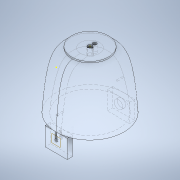
# Autodesk Inventor part: EnclosingRevolver
Saved by Autodesk Inventor 2021.1 (Build 251245010, 245A)
## iProperties
Created: 2023-07-02
Part Number: EnclosingRevolver
Material: ABS Plastic
Document SubType Name: Modeling
Designer: Drake
Density: 1.06 g/cm^3
Appearance: Smooth - White
Author: Drake
Autodesk Inventor part; units mm, degrees
ref_plane "XZ Plane" through (0, 0, 0) normal (0, 1, 0) x (-1, 0, 0)
sketch "Sketch1" plane through (0, 0, 0) normal (0, 1, 0) x (-1, 0, 0)
  arc A0 (-5.4792, -2.4451) -> (-5.4792, 2.4451) centre (0, 0) ccw
  circle A1 centre (0, 0) radius 50
  line L0 (0, 0) -> (0, 6.8)
  circle A2 centre (0, 6.8) radius 0.75
  arc A3 (-5.4792, 2.4451) -> (-5.4792, -2.4451) centre (-6, 0) ccw
  dimension "crescenttop" = 12
  dimension "pantiltmotorholderdiam" = 100
  dimension "screwhole" = 6.8
  dimension "screwhole2" = 1.5
  dimension "CorrectedCrescent" = 5
  constraints: 5 point on circle, 4 centre point, 3 coincident, 2 end point, 1 vertical
  measures "crescenttop" diameter of A0
  measures "pantiltmotorholderdiam" diameter of A1
  measures "screwhole" distance of L0.start L0.end
  measures "screwhole2" diameter of A2
  measures "CorrectedCrescent" diameter of A3
extrude "Extrusion1" add sketch "Sketch1" along normal blind 3.7
ref_plane "Work Plane2" through (-25, 0, 0) normal (1, 0, 0) x (0, 1, 0)
ref_plane "Work Plane1" through (25, 0, 0) normal (1, 0, 0) x (0, 1, 0)
sketch "Sketch3" plane through (0, 0, 0) normal (1, 0, 0) x (0, 1, 0)
  line L0 (0, 25.8902) -> (0, 82.1004) construction
  line L1 (0, 82.1004) -> (-19.2329, 82.1004) construction
  line L2 (-19.2329, 82.1004) -> (-150.2459, 92.0453) construction
  line L3 (-150.2459, 92.0453) -> (-151.1107, 92.0453) construction
  spline S0 degree 4 poles (0, 25.8902) (0, 82.1004) (-19.2329, 82.1004) (-150.2459, 92.0453) (-151.1107, 92.0453) knots 1 1 1 1 1 2 2 2 2 2
  line L4 (0, -50) -> (0, 50) projected
  line L5 (-151.1107, 92.0453) -> (-151.1107, 77.0453)
  line L6 (-151.1107, 77.0453) -> (-80.8125, 71.4468) construction
  line L7 (-80.8125, 71.4468) -> (-20.5383, 53.8321) construction
  line L8 (-20.5383, 53.8321) -> (-22.6717, 53.8321) construction
  line L9 (-22.6717, 53.8321) -> (-15, 0) construction
  spline S1 degree 4 poles (-151.1107, 77.0453) (-80.8125, 71.4468) (-20.5383, 53.8321) (-22.6717, 53.8321) (-15, 0) knots 1 1 1 1 1 2 2 2 2 2
  line L10 (0, 50) -> (0, 0)
  line L11 (0, 50) -> (0, 0)
  line L12 (-15, -28.9058) -> (-15, -27.5917)
  line L13 (0, 25.8902) -> (0, -27.5917)
  line L14 (-15, 0) -> (0, 0)
  dimension "d9" = 15
  dimension "d10" = 15
  constraints: 12 end point, 3 horizontal, 2 point on line, 2 vertical, 1 collinear, 1 parallel, 6 other
  measures "d9" distance of L10.end L9.end
  measures "d10" distance of L3.end L5.end
revolve "Revolution1" add sketch "Sketch3" angle 360 about axis through (0, -15, 0) along (0, -1, 0)
mirror "Mirror1" about plane through (0, 0, 0) normal (0, 0, 1) of "Revolution1"
ref_plane "Work Plane3" through (0, 0, 92.0455) normal (0, 0, 1) x (1, 0, 0)
sketch "Sketch4" plane through (0, 0, 92.0455) normal (0, 0, 1) x (1, 0, 0)
  line L0 (-92.0453, -151.1107) -> (92.0453, -151.1107) projected
  line L1 (-92.0453, -151.1107) -> (-92.0453, -139.1107)
  line L2 (-92.0453, -151.1107) -> (-92.0453, -118.1107)
  line L3 (-92.0453, -118.1107) -> (-92.0453, -113.1107)
  line L4 (-92.0453, -113.1107) -> (0, -113.1107)
  point P0 (0, 0)
  point P1 (0, -151.1107)
  dimension "motorwidth" = 12
  dimension "motorlength" = 33
  dimension "allowance" = 5
  constraints: 8 end point, 3 vertical, 1 coincident, 1 perpendicular
  measures "motorwidth" distance of L0.start L1.end
  measures "motorlength" distance of L0.start L2.end
  measures "allowance" distance of L2.end L3.end
hole "Hole1" at (0, -113.1107, 92.0455) direction (0, 0, -1) diameter 3 end through all
thread "Thread1" size "M3x0.5" class "6H" standard "ANSI Metric M Profile" full length
sketch "Sketch6" plane through (0, -151.1107, 0) normal (0, -1, 0) x (1, 0, 0)
  circle A0 centre (0, 0) radius 92.0453 projected
  circle A1 centre (0, 0) radius 77.0453
  circle A2 centre (0, 0) radius 77.0453 projected
  line L0 (0, -77.0453) -> (25, -77.0453)
  line L1 (25, -77.0453) -> (30, -77.0453)
  line L2 (30, -77.0453) -> (-25, -77.0453)
  line L3 (-25, -77.0453) -> (-30, -77.0453)
  line L4 (-30, -77.0453) -> (-30, -79.5453)
  line L5 (-30, -79.5453) -> (-30, -91.5453)
  line L6 (-30, -91.5453) -> (30, -91.5453)
  line L7 (30, -91.5453) -> (30, -77.0453)
  line L8 (-30, -77.0453) -> (-30, -81.0453)
  point P0 (0, 77.0453)
  point P1 (-4.9974, -76.883)
  point P2 (-4.9974, -91.9095)
  point P3 (0, 92.0453)
  point P4 (4.9974, -91.9095)
  point P5 (-30, -87.0191)
  point P6 (-9.581, -91.5453)
  point P7 (9.581, -91.5453)
  point P8 (30, -87.0191)
  dimension "d43" = 25
  dimension "d44" = 5
  dimension "d45" = 55
  dimension "d46" = 5
  dimension "supportwidth" = 60
  dimension "bushingpenetration" = 2.5
  dimension "d49" = 12
  dimension "d50" = 0
  dimension "d51" = 14.5
  dimension "bushinglength" = 4
  dimension "d60" = 14.5
  constraints: 18 end point, 4 point on line, 3 point on circle, 1 coincident, 1 horizontal, 1 perpendicular, 1 tangent, 1 vertical, 3 other
  measures "d43" distance of L0.start L0.end
  measures "d44" distance of L0.end L1.end
  measures "d45" distance of L1.end L2.end
  measures "d46" distance of L2.end L3.end
  measures "supportwidth" distance of L1.end L3.end
  measures "bushingpenetration" distance of L3.end L4.end
  measures "d49" distance of L4.end L5.end
  measures "d50" angle of L6 L3
  measures "d51" distance from line of L5.end L3
  measures "bushinglength" distance of L3.end L8.end
  measures "d60" distance of L6.end L1.end
extrude "Extrusion2" add sketch "Sketch6" along normal blind 50 contours L5 L4 L3 L2 L0 L1 L7 A0 L6 | A0 L6 L5 | L7 L6 A0
mirror "Mirror2" about plane through (0, 0, 0) normal (0, 0, 1) of "Extrusion2"
sketch "Sketch8" plane through (0, 3.7, 0) normal (0, 1, 0) x (1, 0, 0)
  arc A0 (5.4792, 2.4451) -> (5.4792, -2.4451) centre (0, 0) ccw construction
  line L0 (0, 0) -> (0, 25) construction
  circle A1 centre (0, 0) radius 25 construction
  circle A2 centre (0, 12.5) radius 5
  line L1 (0, 0) -> (0, -6.8)
  circle A3 centre (0, -6.8) radius 0.75
  point P0 (-6, 0)
  point P1 (-6, 0)
  point P2 (-1.4882, 5.8125)
  point P3 (1.4882, 5.8125)
  dimension "d40" = 10
  dimension "d56" = 6.8
  dimension "d57" = 1.5
  constraints: 4 end point, 2 centre point, 2 vertical, 1 coincident, 1 midpoint, 1 vertical alignment, 1 other
  measures "d40" diameter of A2
  measures "d56" distance of L1.start L1.end
  measures "d57" diameter of A3
extrude "Extrusion4" cut sketch "Sketch8" against normal through all
sketch "Sketch9" plane through (0, 3.7, 0) normal (0, 1, 0) x (1, 0, 0)
  point P0 (0, 0)
ref_plane "Work Plane4" through (0, -171.1107, 92.0455) normal (0, 0, 1) x (1, 0, 0)
sketch "Sketch10" plane through (0, -171.1107, 92.0455) normal (0, 0, 1) x (1, 0, 0)
  line L0 (-1.9, 16.6) -> (-2.75, 2.1651)
  line L1 (2.75, 2.1651) -> (1.9, 16.6)
  arc A0 (1.9, 16.6) -> (-1.9, 16.6) centre (0, 16.6) ccw
  circle A1 centre (0, 0) radius 3.5
  circle A2 centre (0, 0) radius 1.25
  line L2 (0.6339, 2.1589) -> (0.3485, 2.4241)
  line L3 (0.3485, 2.4241) -> (0, 2.25)
  line L4 (0, 2.25) -> (-0.3485, 2.4241)
  line L5 (-0.3485, 2.4241) -> (-0.6339, 2.1589)
  line L6 (-0.6339, 2.1589) -> (-1.0174, 2.2278)
  line L7 (-1.0174, 2.2278) -> (-1.2164, 1.8928)
  line L8 (-1.2164, 1.8928) -> (-1.6038, 1.8509)
  line L9 (-1.6038, 1.8509) -> (-1.7004, 1.4734)
  line L10 (-1.7004, 1.4734) -> (-2.0603, 1.3241)
  line L11 (-2.0603, 1.3241) -> (-2.0467, 0.9347)
  line L12 (-2.0467, 0.9347) -> (-2.3499, 0.69)
  line L13 (-2.3499, 0.69) -> (-2.2271, 0.3202)
  line L14 (-2.2271, 0.3202) -> (-2.4491, 0)
  line L15 (-2.4491, 0) -> (-2.2271, -0.3202)
  line L16 (-2.2271, -0.3202) -> (-2.3499, -0.69)
  line L17 (-2.3499, -0.69) -> (-2.0467, -0.9347)
  line L18 (-2.0467, -0.9347) -> (-2.0603, -1.3241)
  line L19 (-2.0603, -1.3241) -> (-1.7004, -1.4734)
  line L20 (-1.7004, -1.4734) -> (-1.6038, -1.8509)
  line L21 (-1.6038, -1.8509) -> (-1.2164, -1.8928)
  line L22 (-1.2164, -1.8928) -> (-1.0174, -2.2278)
  line L23 (-1.0174, -2.2278) -> (-0.6339, -2.1589)
  line L24 (-0.6339, -2.1589) -> (-0.3485, -2.4241)
  line L25 (-0.3485, -2.4241) -> (0, -2.25)
  line L26 (0, -2.25) -> (0.3485, -2.4241)
  line L27 (0.3485, -2.4241) -> (0.6339, -2.1589)
  line L28 (0.6339, -2.1589) -> (1.0174, -2.2278)
  line L29 (1.0174, -2.2278) -> (1.2164, -1.8928)
  line L30 (1.2164, -1.8928) -> (1.6038, -1.8509)
  line L31 (1.6038, -1.8509) -> (1.7004, -1.4734)
  line L32 (1.7004, -1.4734) -> (2.0603, -1.3241)
  line L33 (2.0603, -1.3241) -> (2.0467, -0.9347)
  line L34 (2.0467, -0.9347) -> (2.3499, -0.69)
  line L35 (2.3499, -0.69) -> (2.2271, -0.3202)
  line L36 (2.2271, -0.3202) -> (2.4491, 0)
  line L37 (2.4491, 0) -> (2.2271, 0.3202)
  line L38 (2.2271, 0.3202) -> (2.3499, 0.69)
  line L39 (2.3499, 0.69) -> (2.0467, 0.9347)
  line L40 (2.0467, 0.9347) -> (2.0603, 1.3241)
  line L41 (2.0603, 1.3241) -> (1.7004, 1.4734)
  line L42 (1.7004, 1.4734) -> (1.6038, 1.8509)
  line L43 (1.6038, 1.8509) -> (1.2164, 1.8928)
  line L44 (1.2164, 1.8928) -> (1.0174, 2.2278)
  line L45 (1.0174, 2.2278) -> (0.6339, 2.1589)
  circle A3 centre (0, 0) radius 1.25
  arc A4 (2.75, 2.1651) -> (-2.75, 2.1651) centre (0, 0) ccw
  circle A5 centre (0, 6.8) radius 0.6
  circle A6 centre (0, 8.9) radius 0.6
  circle A7 centre (0, 11) radius 0.6
  circle A8 centre (0, 13.1) radius 0.6
  circle A9 centre (0, 15.2) radius 0.6
  circle A10 centre (0, 17.3) radius 0.6
  point P0 (0, 171.1107)
  constraints: 92 end point, 11 centre point, 4 point on circle, 1 coincident
extrude "Extrusion5" cut sketch "Sketch10" against normal blind 12 contours A0 L1 A1 L0 | A1 | A2 | L45 L44 L43 L42 L41 L40 L39 L38 L37 L36 L35 L34 L33 L32 L31 L30 L29 L28 L27 L26 L25 L24 L23 L22 L21 L20 L19 L18 L17 L16 L15 L14 L13 L12 L11 L10 L9 L8 L7 L6 L5 L4 L3 L2 | A5 | A6 | A7 | A8 | A9 | A10
mirror "Mirror4" [suppressed]
sketch "Sketch11" plane through (0, -171.1107, 80.0455) normal (0, 0, 1) x (1, 0, 0)
  line L0 (-1.9, 16.6) -> (-2.75, 2.1651)
  line L1 (2.75, 2.1651) -> (1.9, 16.6)
  arc A0 (1.9, 16.6) -> (-1.9, 16.6) centre (0, 16.6) ccw
  circle A1 centre (0, 0) radius 3.5
  circle A2 centre (0, 0) radius 1.25
  line L2 (0.6339, 2.1589) -> (0.3485, 2.4241)
  line L3 (0.3485, 2.4241) -> (0, 2.25)
  line L4 (0, 2.25) -> (-0.3485, 2.4241)
  line L5 (-0.3485, 2.4241) -> (-0.6339, 2.1589)
  line L6 (-0.6339, 2.1589) -> (-1.0174, 2.2278)
  line L7 (-1.0174, 2.2278) -> (-1.2164, 1.8928)
  line L8 (-1.2164, 1.8928) -> (-1.6038, 1.8509)
  line L9 (-1.6038, 1.8509) -> (-1.7004, 1.4734)
  line L10 (-1.7004, 1.4734) -> (-2.0603, 1.3241)
  line L11 (-2.0603, 1.3241) -> (-2.0467, 0.9347)
  line L12 (-2.0467, 0.9347) -> (-2.3499, 0.69)
  line L13 (-2.3499, 0.69) -> (-2.2271, 0.3202)
  line L14 (-2.2271, 0.3202) -> (-2.4491, 0)
  line L15 (-2.4491, 0) -> (-2.2271, -0.3202)
  line L16 (-2.2271, -0.3202) -> (-2.3499, -0.69)
  line L17 (-2.3499, -0.69) -> (-2.0467, -0.9347)
  line L18 (-2.0467, -0.9347) -> (-2.0603, -1.3241)
  line L19 (-2.0603, -1.3241) -> (-1.7004, -1.4734)
  line L20 (-1.7004, -1.4734) -> (-1.6038, -1.8509)
  line L21 (-1.6038, -1.8509) -> (-1.2164, -1.8928)
  line L22 (-1.2164, -1.8928) -> (-1.0174, -2.2278)
  line L23 (-1.0174, -2.2278) -> (-0.6339, -2.1589)
  line L24 (-0.6339, -2.1589) -> (-0.3485, -2.4241)
  line L25 (-0.3485, -2.4241) -> (0, -2.25)
  line L26 (0, -2.25) -> (0.3485, -2.4241)
  line L27 (0.3485, -2.4241) -> (0.6339, -2.1589)
  line L28 (0.6339, -2.1589) -> (1.0174, -2.2278)
  line L29 (1.0174, -2.2278) -> (1.2164, -1.8928)
  line L30 (1.2164, -1.8928) -> (1.6038, -1.8509)
  line L31 (1.6038, -1.8509) -> (1.7004, -1.4734)
  line L32 (1.7004, -1.4734) -> (2.0603, -1.3241)
  line L33 (2.0603, -1.3241) -> (2.0467, -0.9347)
  line L34 (2.0467, -0.9347) -> (2.3499, -0.69)
  line L35 (2.3499, -0.69) -> (2.2271, -0.3202)
  line L36 (2.2271, -0.3202) -> (2.4491, 0)
  line L37 (2.4491, 0) -> (2.2271, 0.3202)
  line L38 (2.2271, 0.3202) -> (2.3499, 0.69)
  line L39 (2.3499, 0.69) -> (2.0467, 0.9347)
  line L40 (2.0467, 0.9347) -> (2.0603, 1.3241)
  line L41 (2.0603, 1.3241) -> (1.7004, 1.4734)
  line L42 (1.7004, 1.4734) -> (1.6038, 1.8509)
  line L43 (1.6038, 1.8509) -> (1.2164, 1.8928)
  line L44 (1.2164, 1.8928) -> (1.0174, 2.2278)
  line L45 (1.0174, 2.2278) -> (0.6339, 2.1589)
  circle A3 centre (0, 0) radius 1.25
  arc A4 (2.75, 2.1651) -> (-2.75, 2.1651) centre (0, 0) ccw
  circle A5 centre (0, 6.8) radius 0.6
  circle A6 centre (0, 8.9) radius 0.6
  circle A7 centre (0, 11) radius 0.6
  circle A8 centre (0, 13.1) radius 0.6
  circle A9 centre (0, 15.2) radius 0.6
  circle A10 centre (0, 17.3) radius 0.6
  point P0 (0, 171.1107)
  constraints: 92 end point, 11 centre point, 4 point on circle
extrude "Extrusion6" cut sketch "Sketch11" against normal blind 10 contours A1 | A2 | L45 L44 L43 L42 L41 L40 L39 L38 L37 L36 L35 L34 L33 L32 L31 L30 L29 L28 L27 L26 L25 L24 L23 L22 L21 L20 L19 L18 L17 L16 L15 L14 L13 L12 L11 L10 L9 L8 L7 L6 L5 L4 L3 L2 | A5 | A6 | A7 | A8 | A9 | A10
sketch "Sketch12" plane through (9.581, -151.1107, 91.5453) normal (0, 0, 1) x (1, 0, 0)
  point P0 (-9.581, 151.1107)
mirror "Mirror5" [suppressed]
sketch "Sketch13" plane through (-30, -151.1107, 91.5453) normal (0, 0, 1) x (1, 0, 0)
  point P0 (30, 151.1107)
ref_plane "Work Plane5" through (30, -151.1107, 77.0453) normal (0, 0, 1) x (0, -1, 0)
sketch "Sketch14" plane through (30, -151.1107, 77.0453) normal (0, 0, 1) x (0, -1, 0)
  circle A0 centre (20, -30) radius 1.25
  arc A1 (17.8349, -27.25) -> (17.8349, -32.75) centre (20, -30) ccw projected
  point P0 (-151.1107, -30)
  dimension "bushingholeending" = 2.5
  constraints: 1 centre point, 1 concentric, 2 other
  measures "bushingholeending" diameter of A0
extrude "Extrusion7" [suppressed]
mirror "Mirror6" [suppressed]
sketch "Sketch15" plane through (0, 3.7, 0) normal (0, 1, 0) x (1, 0, 0)
  arc A0 (5.4792, 2.4451) -> (5.4792, -2.4451) centre (0, 0) ccw projected
  arc A1 (1.4882, 5.8125) -> (0, 7.5) centre (0, 6) ccw projected
  arc A2 (0, 7.5) -> (-1.4882, 5.8125) centre (0, 6) ccw projected
  arc A3 (5.4792, -2.4451) -> (5.4792, 2.4451) centre (6, 0) ccw projected
  dimension "d71" = 6
  dimension "d72" = 2.5
  measures "d71" radius of A0
  measures "d72" radius of A3
extrude "Extrusion8" cut sketch "Sketch15" against normal through all contours A3 A0
sketch "Sketch16" plane through (30, -151.1107, -91.5453) normal (0, 0, -1) x (-1, 0, 0)
  arc A0 (27.25, -17.8349) -> (32.75, -17.8349) centre (30, -20) ccw projected
  circle A1 centre (30, -20) radius 21.5
  point P0 (30, 151.1107)
  dimension "bearing" = 43
  constraints: 1 centre point, 1 coincident
  measures "bearing" diameter of A1
extrude "Extrusion9" [suppressed]
sketch "Sketch17" plane through (-30, -201.1107, -77.0453) normal (0, 0, 1) x (1, 0, 0)
  arc A0 (22.1101, 50) -> (37.8899, 50) centre (30, 30) ccw projected
  circle A1 centre (30, 30) radius 11.5
  point P0 (30, 201.1107)
  dimension "bearingouterdiam" = 23
  constraints: 1 centre point, 1 coincident, 1 horizontal alignment
  measures "bearingouterdiam" diameter of A1
extrude "Extrusion10" cut sketch "Sketch17" against normal blind 8
equation "\"d57\" = screwhole2"
body "Solid1"
